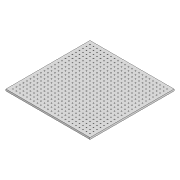
# Autodesk Inventor part: opticalPlate
Saved by Autodesk Inventor 2021 (Build 250183000, 183)
## iProperties
Created: 2020-10-05
Part Number: opticalPlate
Material: Generic
Document SubType Name: Modeling
Designer: Derm
Density: 1 g/cm^3
Appearance: Default
Author: Derm
Autodesk Inventor part; units mm, degrees
ref_plane "YZ Plane" through (0, 0, 0) normal (1, 0, 0) x (0, 1, 0)
ref_plane "XZ Plane" through (0, 0, 0) normal (0, 1, 0) x (-1, 0, 0)
ref_plane "XY Plane" through (0, 0, 0) normal (0, 0, 1) x (1, 0, 0)
sketch "Sketch1" plane through (0, 0, 0) normal (0, 1, 0) x (-1, 0, 0)
  line L0 (0, 0) -> (609.6, 0)
  line L1 (609.6, 0) -> (609.6, -609.6)
  line L2 (609.6, -609.6) -> (0, -609.6)
  line L3 (0, -609.6) -> (0, 0)
  circle A0 centre (25.4, -25.4) radius 3.175
  circle A1 centre (50.8, -25.4) radius 3.175
  circle A2 centre (76.2, -25.4) radius 3.175
  circle A3 centre (101.6, -25.4) radius 3.175
  circle A4 centre (127, -25.4) radius 3.175
  circle A5 centre (152.4, -25.4) radius 3.175
  circle A6 centre (177.8, -25.4) radius 3.175
  circle A7 centre (203.2, -25.4) radius 3.175
  circle A8 centre (228.6, -25.4) radius 3.175
  circle A9 centre (254, -25.4) radius 3.175
  circle A10 centre (279.4, -25.4) radius 3.175
  circle A11 centre (304.8, -25.4) radius 3.175
  circle A12 centre (330.2, -25.4) radius 3.175
  circle A13 centre (355.6, -25.4) radius 3.175
  circle A14 centre (381, -25.4) radius 3.175
  circle A15 centre (406.4, -25.4) radius 3.175
  circle A16 centre (431.8, -25.4) radius 3.175
  circle A17 centre (457.2, -25.4) radius 3.175
  circle A18 centre (482.6, -25.4) radius 3.175
  circle A19 centre (508, -25.4) radius 3.175
  circle A20 centre (533.4, -25.4) radius 3.175
  circle A21 centre (558.8, -25.4) radius 3.175
  circle A22 centre (584.2, -25.4) radius 3.175
  circle A23 centre (25.4, -50.8) radius 3.175
  circle A24 centre (50.8, -50.8) radius 3.175
  circle A25 centre (76.2, -50.8) radius 3.175
  circle A26 centre (101.6, -50.8) radius 3.175
  circle A27 centre (127, -50.8) radius 3.175
  circle A28 centre (152.4, -50.8) radius 3.175
  circle A29 centre (177.8, -50.8) radius 3.175
  circle A30 centre (203.2, -50.8) radius 3.175
  circle A31 centre (228.6, -50.8) radius 3.175
  circle A32 centre (254, -50.8) radius 3.175
  circle A33 centre (279.4, -50.8) radius 3.175
  circle A34 centre (304.8, -50.8) radius 3.175
  circle A35 centre (330.2, -50.8) radius 3.175
  circle A36 centre (355.6, -50.8) radius 3.175
  circle A37 centre (381, -50.8) radius 3.175
  circle A38 centre (406.4, -50.8) radius 3.175
  circle A39 centre (431.8, -50.8) radius 3.175
  circle A40 centre (457.2, -50.8) radius 3.175
  circle A41 centre (482.6, -50.8) radius 3.175
  circle A42 centre (508, -50.8) radius 3.175
  circle A43 centre (533.4, -50.8) radius 3.175
  circle A44 centre (558.8, -50.8) radius 3.175
  circle A45 centre (584.2, -50.8) radius 3.175
  circle A46 centre (25.4, -76.2) radius 3.175
  circle A47 centre (50.8, -76.2) radius 3.175
  circle A48 centre (76.2, -76.2) radius 3.175
  circle A49 centre (101.6, -76.2) radius 3.175
  circle A50 centre (127, -76.2) radius 3.175
  circle A51 centre (152.4, -76.2) radius 3.175
  circle A52 centre (177.8, -76.2) radius 3.175
  circle A53 centre (203.2, -76.2) radius 3.175
  circle A54 centre (228.6, -76.2) radius 3.175
  circle A55 centre (254, -76.2) radius 3.175
  circle A56 centre (279.4, -76.2) radius 3.175
  circle A57 centre (304.8, -76.2) radius 3.175
  circle A58 centre (330.2, -76.2) radius 3.175
  circle A59 centre (355.6, -76.2) radius 3.175
  circle A60 centre (381, -76.2) radius 3.175
  circle A61 centre (406.4, -76.2) radius 3.175
  circle A62 centre (431.8, -76.2) radius 3.175
  circle A63 centre (457.2, -76.2) radius 3.175
  circle A64 centre (482.6, -76.2) radius 3.175
  circle A65 centre (508, -76.2) radius 3.175
  circle A66 centre (533.4, -76.2) radius 3.175
  circle A67 centre (558.8, -76.2) radius 3.175
  circle A68 centre (584.2, -76.2) radius 3.175
  circle A69 centre (25.4, -101.6) radius 3.175
  circle A70 centre (50.8, -101.6) radius 3.175
  circle A71 centre (76.2, -101.6) radius 3.175
  circle A72 centre (101.6, -101.6) radius 3.175
  circle A73 centre (127, -101.6) radius 3.175
  circle A74 centre (152.4, -101.6) radius 3.175
  circle A75 centre (177.8, -101.6) radius 3.175
  circle A76 centre (203.2, -101.6) radius 3.175
  circle A77 centre (228.6, -101.6) radius 3.175
  circle A78 centre (254, -101.6) radius 3.175
  circle A79 centre (279.4, -101.6) radius 3.175
  circle A80 centre (304.8, -101.6) radius 3.175
  circle A81 centre (330.2, -101.6) radius 3.175
  circle A82 centre (355.6, -101.6) radius 3.175
  circle A83 centre (381, -101.6) radius 3.175
  circle A84 centre (406.4, -101.6) radius 3.175
  circle A85 centre (431.8, -101.6) radius 3.175
  circle A86 centre (457.2, -101.6) radius 3.175
  circle A87 centre (482.6, -101.6) radius 3.175
  circle A88 centre (508, -101.6) radius 3.175
  circle A89 centre (533.4, -101.6) radius 3.175
  circle A90 centre (558.8, -101.6) radius 3.175
  circle A91 centre (584.2, -101.6) radius 3.175
  circle A92 centre (25.4, -127) radius 3.175
  circle A93 centre (50.8, -127) radius 3.175
  circle A94 centre (76.2, -127) radius 3.175
  circle A95 centre (101.6, -127) radius 3.175
  circle A96 centre (127, -127) radius 3.175
  circle A97 centre (152.4, -127) radius 3.175
  circle A98 centre (177.8, -127) radius 3.175
  circle A99 centre (203.2, -127) radius 3.175
  circle A100 centre (228.6, -127) radius 3.175
  circle A101 centre (254, -127) radius 3.175
  circle A102 centre (279.4, -127) radius 3.175
  circle A103 centre (304.8, -127) radius 3.175
  circle A104 centre (330.2, -127) radius 3.175
  circle A105 centre (355.6, -127) radius 3.175
  circle A106 centre (381, -127) radius 3.175
  circle A107 centre (406.4, -127) radius 3.175
  circle A108 centre (431.8, -127) radius 3.175
  circle A109 centre (457.2, -127) radius 3.175
  circle A110 centre (482.6, -127) radius 3.175
  circle A111 centre (508, -127) radius 3.175
  circle A112 centre (533.4, -127) radius 3.175
  circle A113 centre (558.8, -127) radius 3.175
  circle A114 centre (584.2, -127) radius 3.175
  circle A115 centre (25.4, -152.4) radius 3.175
  circle A116 centre (50.8, -152.4) radius 3.175
  circle A117 centre (76.2, -152.4) radius 3.175
  circle A118 centre (101.6, -152.4) radius 3.175
  circle A119 centre (127, -152.4) radius 3.175
  circle A120 centre (152.4, -152.4) radius 3.175
  circle A121 centre (177.8, -152.4) radius 3.175
  circle A122 centre (203.2, -152.4) radius 3.175
  circle A123 centre (228.6, -152.4) radius 3.175
  circle A124 centre (254, -152.4) radius 3.175
  circle A125 centre (279.4, -152.4) radius 3.175
  circle A126 centre (304.8, -152.4) radius 3.175
  circle A127 centre (330.2, -152.4) radius 3.175
  circle A128 centre (355.6, -152.4) radius 3.175
  circle A129 centre (381, -152.4) radius 3.175
  circle A130 centre (406.4, -152.4) radius 3.175
  circle A131 centre (431.8, -152.4) radius 3.175
  circle A132 centre (457.2, -152.4) radius 3.175
  circle A133 centre (482.6, -152.4) radius 3.175
  circle A134 centre (508, -152.4) radius 3.175
  circle A135 centre (533.4, -152.4) radius 3.175
  circle A136 centre (558.8, -152.4) radius 3.175
  circle A137 centre (584.2, -152.4) radius 3.175
  circle A138 centre (25.4, -177.8) radius 3.175
  circle A139 centre (50.8, -177.8) radius 3.175
  circle A140 centre (76.2, -177.8) radius 3.175
  circle A141 centre (101.6, -177.8) radius 3.175
  circle A142 centre (127, -177.8) radius 3.175
  circle A143 centre (152.4, -177.8) radius 3.175
  circle A144 centre (177.8, -177.8) radius 3.175
  circle A145 centre (203.2, -177.8) radius 3.175
  circle A146 centre (228.6, -177.8) radius 3.175
  circle A147 centre (254, -177.8) radius 3.175
  circle A148 centre (279.4, -177.8) radius 3.175
  circle A149 centre (304.8, -177.8) radius 3.175
  circle A150 centre (330.2, -177.8) radius 3.175
  circle A151 centre (355.6, -177.8) radius 3.175
  circle A152 centre (381, -177.8) radius 3.175
  circle A153 centre (406.4, -177.8) radius 3.175
  circle A154 centre (431.8, -177.8) radius 3.175
  circle A155 centre (457.2, -177.8) radius 3.175
  circle A156 centre (482.6, -177.8) radius 3.175
  circle A157 centre (508, -177.8) radius 3.175
  circle A158 centre (533.4, -177.8) radius 3.175
  circle A159 centre (558.8, -177.8) radius 3.175
  circle A160 centre (584.2, -177.8) radius 3.175
  circle A161 centre (25.4, -203.2) radius 3.175
  circle A162 centre (50.8, -203.2) radius 3.175
  circle A163 centre (76.2, -203.2) radius 3.175
  circle A164 centre (101.6, -203.2) radius 3.175
  circle A165 centre (127, -203.2) radius 3.175
  circle A166 centre (152.4, -203.2) radius 3.175
  circle A167 centre (177.8, -203.2) radius 3.175
  circle A168 centre (203.2, -203.2) radius 3.175
  circle A169 centre (228.6, -203.2) radius 3.175
  circle A170 centre (254, -203.2) radius 3.175
  circle A171 centre (279.4, -203.2) radius 3.175
  circle A172 centre (304.8, -203.2) radius 3.175
  circle A173 centre (330.2, -203.2) radius 3.175
  circle A174 centre (355.6, -203.2) radius 3.175
  circle A175 centre (381, -203.2) radius 3.175
  circle A176 centre (406.4, -203.2) radius 3.175
  circle A177 centre (431.8, -203.2) radius 3.175
  circle A178 centre (457.2, -203.2) radius 3.175
  circle A179 centre (482.6, -203.2) radius 3.175
  circle A180 centre (508, -203.2) radius 3.175
  circle A181 centre (533.4, -203.2) radius 3.175
  circle A182 centre (558.8, -203.2) radius 3.175
  circle A183 centre (584.2, -203.2) radius 3.175
  circle A184 centre (25.4, -228.6) radius 3.175
  circle A185 centre (50.8, -228.6) radius 3.175
  circle A186 centre (76.2, -228.6) radius 3.175
  circle A187 centre (101.6, -228.6) radius 3.175
  circle A188 centre (127, -228.6) radius 3.175
  circle A189 centre (152.4, -228.6) radius 3.175
  circle A190 centre (177.8, -228.6) radius 3.175
  circle A191 centre (203.2, -228.6) radius 3.175
  circle A192 centre (228.6, -228.6) radius 3.175
  circle A193 centre (254, -228.6) radius 3.175
  circle A194 centre (279.4, -228.6) radius 3.175
  circle A195 centre (304.8, -228.6) radius 3.175
  circle A196 centre (330.2, -228.6) radius 3.175
  circle A197 centre (355.6, -228.6) radius 3.175
  circle A198 centre (381, -228.6) radius 3.175
  circle A199 centre (406.4, -228.6) radius 3.175
  circle A200 centre (431.8, -228.6) radius 3.175
  circle A201 centre (457.2, -228.6) radius 3.175
  circle A202 centre (482.6, -228.6) radius 3.175
  circle A203 centre (508, -228.6) radius 3.175
  circle A204 centre (533.4, -228.6) radius 3.175
  circle A205 centre (558.8, -228.6) radius 3.175
  circle A206 centre (584.2, -228.6) radius 3.175
  circle A207 centre (25.4, -254) radius 3.175
  circle A208 centre (50.8, -254) radius 3.175
  circle A209 centre (76.2, -254) radius 3.175
  circle A210 centre (101.6, -254) radius 3.175
  circle A211 centre (127, -254) radius 3.175
  circle A212 centre (152.4, -254) radius 3.175
  circle A213 centre (177.8, -254) radius 3.175
  circle A214 centre (203.2, -254) radius 3.175
  circle A215 centre (228.6, -254) radius 3.175
  circle A216 centre (254, -254) radius 3.175
  circle A217 centre (279.4, -254) radius 3.175
  circle A218 centre (304.8, -254) radius 3.175
  circle A219 centre (330.2, -254) radius 3.175
  circle A220 centre (355.6, -254) radius 3.175
  circle A221 centre (381, -254) radius 3.175
  circle A222 centre (406.4, -254) radius 3.175
  circle A223 centre (431.8, -254) radius 3.175
  circle A224 centre (457.2, -254) radius 3.175
  circle A225 centre (482.6, -254) radius 3.175
  circle A226 centre (508, -254) radius 3.175
  circle A227 centre (533.4, -254) radius 3.175
  circle A228 centre (558.8, -254) radius 3.175
  circle A229 centre (584.2, -254) radius 3.175
  circle A230 centre (25.4, -279.4) radius 3.175
  circle A231 centre (50.8, -279.4) radius 3.175
  circle A232 centre (76.2, -279.4) radius 3.175
  circle A233 centre (101.6, -279.4) radius 3.175
  circle A234 centre (127, -279.4) radius 3.175
  circle A235 centre (152.4, -279.4) radius 3.175
  circle A236 centre (177.8, -279.4) radius 3.175
  circle A237 centre (203.2, -279.4) radius 3.175
  circle A238 centre (228.6, -279.4) radius 3.175
  circle A239 centre (254, -279.4) radius 3.175
  circle A240 centre (279.4, -279.4) radius 3.175
  circle A241 centre (304.8, -279.4) radius 3.175
  circle A242 centre (330.2, -279.4) radius 3.175
  circle A243 centre (355.6, -279.4) radius 3.175
  circle A244 centre (381, -279.4) radius 3.175
  circle A245 centre (406.4, -279.4) radius 3.175
  circle A246 centre (431.8, -279.4) radius 3.175
  circle A247 centre (457.2, -279.4) radius 3.175
  circle A248 centre (482.6, -279.4) radius 3.175
  circle A249 centre (508, -279.4) radius 3.175
  circle A250 centre (533.4, -279.4) radius 3.175
  circle A251 centre (558.8, -279.4) radius 3.175
  circle A252 centre (584.2, -279.4) radius 3.175
  circle A253 centre (25.4, -304.8) radius 3.175
  circle A254 centre (50.8, -304.8) radius 3.175
  circle A255 centre (76.2, -304.8) radius 3.175
  circle A256 centre (101.6, -304.8) radius 3.175
  circle A257 centre (127, -304.8) radius 3.175
  circle A258 centre (152.4, -304.8) radius 3.175
  circle A259 centre (177.8, -304.8) radius 3.175
  circle A260 centre (203.2, -304.8) radius 3.175
  circle A261 centre (228.6, -304.8) radius 3.175
  circle A262 centre (254, -304.8) radius 3.175
  circle A263 centre (279.4, -304.8) radius 3.175
  circle A264 centre (304.8, -304.8) radius 3.175
  circle A265 centre (330.2, -304.8) radius 3.175
  circle A266 centre (355.6, -304.8) radius 3.175
  circle A267 centre (381, -304.8) radius 3.175
  circle A268 centre (406.4, -304.8) radius 3.175
  circle A269 centre (431.8, -304.8) radius 3.175
  circle A270 centre (457.2, -304.8) radius 3.175
  circle A271 centre (482.6, -304.8) radius 3.175
  circle A272 centre (508, -304.8) radius 3.175
  circle A273 centre (533.4, -304.8) radius 3.175
  circle A274 centre (558.8, -304.8) radius 3.175
  circle A275 centre (584.2, -304.8) radius 3.175
  circle A276 centre (25.4, -330.2) radius 3.175
  circle A277 centre (50.8, -330.2) radius 3.175
  circle A278 centre (76.2, -330.2) radius 3.175
  circle A279 centre (101.6, -330.2) radius 3.175
  circle A280 centre (127, -330.2) radius 3.175
  circle A281 centre (152.4, -330.2) radius 3.175
  circle A282 centre (177.8, -330.2) radius 3.175
  circle A283 centre (203.2, -330.2) radius 3.175
  circle A284 centre (228.6, -330.2) radius 3.175
  circle A285 centre (254, -330.2) radius 3.175
  circle A286 centre (279.4, -330.2) radius 3.175
  circle A287 centre (304.8, -330.2) radius 3.175
  circle A288 centre (330.2, -330.2) radius 3.175
  circle A289 centre (355.6, -330.2) radius 3.175
  circle A290 centre (381, -330.2) radius 3.175
  circle A291 centre (406.4, -330.2) radius 3.175
  circle A292 centre (431.8, -330.2) radius 3.175
  circle A293 centre (457.2, -330.2) radius 3.175
  circle A294 centre (482.6, -330.2) radius 3.175
  circle A295 centre (508, -330.2) radius 3.175
  circle A296 centre (533.4, -330.2) radius 3.175
  circle A297 centre (558.8, -330.2) radius 3.175
  circle A298 centre (584.2, -330.2) radius 3.175
  circle A299 centre (25.4, -355.6) radius 3.175
  circle A300 centre (50.8, -355.6) radius 3.175
  circle A301 centre (76.2, -355.6) radius 3.175
  circle A302 centre (101.6, -355.6) radius 3.175
  circle A303 centre (127, -355.6) radius 3.175
  circle A304 centre (152.4, -355.6) radius 3.175
  circle A305 centre (177.8, -355.6) radius 3.175
  circle A306 centre (203.2, -355.6) radius 3.175
  circle A307 centre (228.6, -355.6) radius 3.175
  circle A308 centre (254, -355.6) radius 3.175
  circle A309 centre (279.4, -355.6) radius 3.175
  circle A310 centre (304.8, -355.6) radius 3.175
  circle A311 centre (330.2, -355.6) radius 3.175
  circle A312 centre (355.6, -355.6) radius 3.175
  circle A313 centre (381, -355.6) radius 3.175
  circle A314 centre (406.4, -355.6) radius 3.175
  circle A315 centre (431.8, -355.6) radius 3.175
  circle A316 centre (457.2, -355.6) radius 3.175
  circle A317 centre (482.6, -355.6) radius 3.175
  circle A318 centre (508, -355.6) radius 3.175
  circle A319 centre (533.4, -355.6) radius 3.175
  circle A320 centre (558.8, -355.6) radius 3.175
  circle A321 centre (584.2, -355.6) radius 3.175
  circle A322 centre (25.4, -381) radius 3.175
  circle A323 centre (50.8, -381) radius 3.175
  circle A324 centre (76.2, -381) radius 3.175
  circle A325 centre (101.6, -381) radius 3.175
  circle A326 centre (127, -381) radius 3.175
  circle A327 centre (152.4, -381) radius 3.175
  circle A328 centre (177.8, -381) radius 3.175
  circle A329 centre (203.2, -381) radius 3.175
  circle A330 centre (228.6, -381) radius 3.175
  circle A331 centre (254, -381) radius 3.175
  circle A332 centre (279.4, -381) radius 3.175
  circle A333 centre (304.8, -381) radius 3.175
  circle A334 centre (330.2, -381) radius 3.175
  circle A335 centre (355.6, -381) radius 3.175
  circle A336 centre (381, -381) radius 3.175
  circle A337 centre (406.4, -381) radius 3.175
  circle A338 centre (431.8, -381) radius 3.175
  circle A339 centre (457.2, -381) radius 3.175
  circle A340 centre (482.6, -381) radius 3.175
  circle A341 centre (508, -381) radius 3.175
  circle A342 centre (533.4, -381) radius 3.175
  circle A343 centre (558.8, -381) radius 3.175
  circle A344 centre (584.2, -381) radius 3.175
  circle A345 centre (25.4, -406.4) radius 3.175
  circle A346 centre (50.8, -406.4) radius 3.175
  circle A347 centre (76.2, -406.4) radius 3.175
  circle A348 centre (101.6, -406.4) radius 3.175
  circle A349 centre (127, -406.4) radius 3.175
  circle A350 centre (152.4, -406.4) radius 3.175
  circle A351 centre (177.8, -406.4) radius 3.175
  circle A352 centre (203.2, -406.4) radius 3.175
  circle A353 centre (228.6, -406.4) radius 3.175
  circle A354 centre (254, -406.4) radius 3.175
  circle A355 centre (279.4, -406.4) radius 3.175
  circle A356 centre (304.8, -406.4) radius 3.175
  circle A357 centre (330.2, -406.4) radius 3.175
  circle A358 centre (355.6, -406.4) radius 3.175
  circle A359 centre (381, -406.4) radius 3.175
  circle A360 centre (406.4, -406.4) radius 3.175
  circle A361 centre (431.8, -406.4) radius 3.175
  circle A362 centre (457.2, -406.4) radius 3.175
  circle A363 centre (482.6, -406.4) radius 3.175
  circle A364 centre (508, -406.4) radius 3.175
  circle A365 centre (533.4, -406.4) radius 3.175
  circle A366 centre (558.8, -406.4) radius 3.175
  circle A367 centre (584.2, -406.4) radius 3.175
  circle A368 centre (25.4, -431.8) radius 3.175
  circle A369 centre (50.8, -431.8) radius 3.175
  circle A370 centre (76.2, -431.8) radius 3.175
  circle A371 centre (101.6, -431.8) radius 3.175
  circle A372 centre (127, -431.8) radius 3.175
  circle A373 centre (152.4, -431.8) radius 3.175
  circle A374 centre (177.8, -431.8) radius 3.175
  circle A375 centre (203.2, -431.8) radius 3.175
  circle A376 centre (228.6, -431.8) radius 3.175
  circle A377 centre (254, -431.8) radius 3.175
  circle A378 centre (279.4, -431.8) radius 3.175
  circle A379 centre (304.8, -431.8) radius 3.175
  circle A380 centre (330.2, -431.8) radius 3.175
  circle A381 centre (355.6, -431.8) radius 3.175
  circle A382 centre (381, -431.8) radius 3.175
  circle A383 centre (406.4, -431.8) radius 3.175
  circle A384 centre (431.8, -431.8) radius 3.175
  circle A385 centre (457.2, -431.8) radius 3.175
  circle A386 centre (482.6, -431.8) radius 3.175
  circle A387 centre (508, -431.8) radius 3.175
  circle A388 centre (533.4, -431.8) radius 3.175
  circle A389 centre (558.8, -431.8) radius 3.175
  circle A390 centre (584.2, -431.8) radius 3.175
  circle A391 centre (25.4, -457.2) radius 3.175
  circle A392 centre (50.8, -457.2) radius 3.175
  circle A393 centre (76.2, -457.2) radius 3.175
  circle A394 centre (101.6, -457.2) radius 3.175
  circle A395 centre (127, -457.2) radius 3.175
  circle A396 centre (152.4, -457.2) radius 3.175
  circle A397 centre (177.8, -457.2) radius 3.175
  circle A398 centre (203.2, -457.2) radius 3.175
  circle A399 centre (228.6, -457.2) radius 3.175
  circle A400 centre (254, -457.2) radius 3.175
  circle A401 centre (279.4, -457.2) radius 3.175
  circle A402 centre (304.8, -457.2) radius 3.175
  circle A403 centre (330.2, -457.2) radius 3.175
  circle A404 centre (355.6, -457.2) radius 3.175
  circle A405 centre (381, -457.2) radius 3.175
  circle A406 centre (406.4, -457.2) radius 3.175
  circle A407 centre (431.8, -457.2) radius 3.175
  circle A408 centre (457.2, -457.2) radius 3.175
  circle A409 centre (482.6, -457.2) radius 3.175
  circle A410 centre (508, -457.2) radius 3.175
  circle A411 centre (533.4, -457.2) radius 3.175
  circle A412 centre (558.8, -457.2) radius 3.175
  circle A413 centre (584.2, -457.2) radius 3.175
  circle A414 centre (25.4, -482.6) radius 3.175
  circle A415 centre (50.8, -482.6) radius 3.175
  circle A416 centre (76.2, -482.6) radius 3.175
  circle A417 centre (101.6, -482.6) radius 3.175
  circle A418 centre (127, -482.6) radius 3.175
  circle A419 centre (152.4, -482.6) radius 3.175
  circle A420 centre (177.8, -482.6) radius 3.175
  circle A421 centre (203.2, -482.6) radius 3.175
  circle A422 centre (228.6, -482.6) radius 3.175
  circle A423 centre (254, -482.6) radius 3.175
  circle A424 centre (279.4, -482.6) radius 3.175
  circle A425 centre (304.8, -482.6) radius 3.175
  circle A426 centre (330.2, -482.6) radius 3.175
  circle A427 centre (355.6, -482.6) radius 3.175
  circle A428 centre (381, -482.6) radius 3.175
  circle A429 centre (406.4, -482.6) radius 3.175
  circle A430 centre (431.8, -482.6) radius 3.175
  circle A431 centre (457.2, -482.6) radius 3.175
  circle A432 centre (482.6, -482.6) radius 3.175
  circle A433 centre (508, -482.6) radius 3.175
  circle A434 centre (533.4, -482.6) radius 3.175
  circle A435 centre (558.8, -482.6) radius 3.175
  circle A436 centre (584.2, -482.6) radius 3.175
  circle A437 centre (25.4, -508) radius 3.175
  circle A438 centre (50.8, -508) radius 3.175
  circle A439 centre (76.2, -508) radius 3.175
  circle A440 centre (101.6, -508) radius 3.175
  circle A441 centre (127, -508) radius 3.175
  circle A442 centre (152.4, -508) radius 3.175
  circle A443 centre (177.8, -508) radius 3.175
  circle A444 centre (203.2, -508) radius 3.175
  circle A445 centre (228.6, -508) radius 3.175
  circle A446 centre (254, -508) radius 3.175
  circle A447 centre (279.4, -508) radius 3.175
  circle A448 centre (304.8, -508) radius 3.175
  circle A449 centre (330.2, -508) radius 3.175
  circle A450 centre (355.6, -508) radius 3.175
  circle A451 centre (381, -508) radius 3.175
  circle A452 centre (406.4, -508) radius 3.175
  circle A453 centre (431.8, -508) radius 3.175
  circle A454 centre (457.2, -508) radius 3.175
  circle A455 centre (482.6, -508) radius 3.175
  circle A456 centre (508, -508) radius 3.175
  circle A457 centre (533.4, -508) radius 3.175
  circle A458 centre (558.8, -508) radius 3.175
  circle A459 centre (584.2, -508) radius 3.175
  circle A460 centre (25.4, -533.4) radius 3.175
  circle A461 centre (50.8, -533.4) radius 3.175
  circle A462 centre (76.2, -533.4) radius 3.175
  circle A463 centre (101.6, -533.4) radius 3.175
  circle A464 centre (127, -533.4) radius 3.175
  circle A465 centre (152.4, -533.4) radius 3.175
  circle A466 centre (177.8, -533.4) radius 3.175
  circle A467 centre (203.2, -533.4) radius 3.175
  circle A468 centre (228.6, -533.4) radius 3.175
  circle A469 centre (254, -533.4) radius 3.175
  circle A470 centre (279.4, -533.4) radius 3.175
  circle A471 centre (304.8, -533.4) radius 3.175
  circle A472 centre (330.2, -533.4) radius 3.175
  circle A473 centre (355.6, -533.4) radius 3.175
  circle A474 centre (381, -533.4) radius 3.175
  circle A475 centre (406.4, -533.4) radius 3.175
  circle A476 centre (431.8, -533.4) radius 3.175
  circle A477 centre (457.2, -533.4) radius 3.175
  circle A478 centre (482.6, -533.4) radius 3.175
  circle A479 centre (508, -533.4) radius 3.175
  circle A480 centre (533.4, -533.4) radius 3.175
  circle A481 centre (558.8, -533.4) radius 3.175
  circle A482 centre (584.2, -533.4) radius 3.175
  circle A483 centre (25.4, -558.8) radius 3.175
  circle A484 centre (50.8, -558.8) radius 3.175
  circle A485 centre (76.2, -558.8) radius 3.175
  circle A486 centre (101.6, -558.8) radius 3.175
  circle A487 centre (127, -558.8) radius 3.175
  circle A488 centre (152.4, -558.8) radius 3.175
  circle A489 centre (177.8, -558.8) radius 3.175
  circle A490 centre (203.2, -558.8) radius 3.175
  circle A491 centre (228.6, -558.8) radius 3.175
  circle A492 centre (254, -558.8) radius 3.175
  circle A493 centre (279.4, -558.8) radius 3.175
  circle A494 centre (304.8, -558.8) radius 3.175
  circle A495 centre (330.2, -558.8) radius 3.175
  circle A496 centre (355.6, -558.8) radius 3.175
  circle A497 centre (381, -558.8) radius 3.175
  circle A498 centre (406.4, -558.8) radius 3.175
  circle A499 centre (431.8, -558.8) radius 3.175
  circle A500 centre (457.2, -558.8) radius 3.175
  circle A501 centre (482.6, -558.8) radius 3.175
  circle A502 centre (508, -558.8) radius 3.175
  circle A503 centre (533.4, -558.8) radius 3.175
  circle A504 centre (558.8, -558.8) radius 3.175
  circle A505 centre (584.2, -558.8) radius 3.175
  circle A506 centre (25.4, -584.2) radius 3.175
  circle A507 centre (50.8, -584.2) radius 3.175
  circle A508 centre (76.2, -584.2) radius 3.175
  circle A509 centre (101.6, -584.2) radius 3.175
  circle A510 centre (127, -584.2) radius 3.175
  circle A511 centre (152.4, -584.2) radius 3.175
  circle A512 centre (177.8, -584.2) radius 3.175
  circle A513 centre (203.2, -584.2) radius 3.175
  circle A514 centre (228.6, -584.2) radius 3.175
  circle A515 centre (254, -584.2) radius 3.175
  circle A516 centre (279.4, -584.2) radius 3.175
  circle A517 centre (304.8, -584.2) radius 3.175
  circle A518 centre (330.2, -584.2) radius 3.175
  circle A519 centre (355.6, -584.2) radius 3.175
  circle A520 centre (381, -584.2) radius 3.175
  circle A521 centre (406.4, -584.2) radius 3.175
  circle A522 centre (431.8, -584.2) radius 3.175
  circle A523 centre (457.2, -584.2) radius 3.175
  circle A524 centre (482.6, -584.2) radius 3.175
  circle A525 centre (508, -584.2) radius 3.175
  circle A526 centre (533.4, -584.2) radius 3.175
  circle A527 centre (558.8, -584.2) radius 3.175
  circle A528 centre (584.2, -584.2) radius 3.175
  dimension "d0" = 609.6
  dimension "d1" = 609.6
  dimension "d2" = 6.35
  dimension "d3" = 25.4
  dimension "d4" = 25.4
  dimension "d7" = 25.4
  dimension "d10" = 25.4
  constraints: 529 centre point, 8 end point, 2 horizontal, 2 parallel, 1 perpendicular, 1 vertical, 1056 other
  measures "d0" distance of L0.end L1.end
  measures "d1" distance of L1.end L2.end
  measures "d2" diameter of A0
  measures "d3" distance from line of L3 A0.centre
  measures "d4" distance from line of L0 A0.centre
  measures "d7" distance of A0.centre A1.centre
  measures "d10" distance of A0.centre A23.centre
extrude "Extrusion1" add sketch "Sketch1" along normal blind 12.7
body "Solid1"
